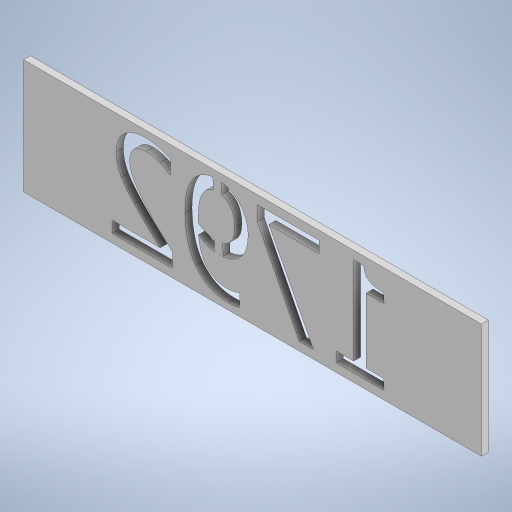
# Autodesk Inventor part: 1792 plate
Saved by Autodesk Inventor 2023.4 (Build 274418000, 418)
## iProperties
Created: 2023-12-26
Part Number: 1792 plate
Material: Generic
Document SubType Name: Sheet Metal
Designer: amrom
Density: 1 g/cm^3
Sheet Metal Rule: Default
Appearance: Default
Author: amrom
Autodesk Inventor part; units mm, degrees
ref_plane "YZ Plane" through (0, 0, 0) normal (1, 0, 0) x (0, 1, 0)
ref_plane "XZ Plane" through (0, 0, 0) normal (0, 1, 0) x (-1, 0, 0)
ref_plane "XY Plane" through (0, 0, 0) normal (0, 0, 1) x (1, 0, 0)
sketch "Sketch1" plane through (0, 0, 0) normal (0, 0, 1) x (1, 0, 0)
  line L0 (0, 0) -> (203.2, 0)
  line L1 (203.2, 0) -> (203.2, 50.8)
  line L2 (203.2, 50.8) -> (0, 50.8)
  line L3 (0, 50.8) -> (0, 0)
  dimension "d0" = 203.2
  dimension "d1" = 50.8
  measures "d0" distance of L2.end L1.end
  measures "d1" distance of L0.end L1.end
extrude "Plate1" add sketch "Sketch1" along normal blind 3.048
sketch "Sketch2" plane through (0, 0, 0) normal (0, 0, -1) x (-1, 0, 0)
  line L0 (-203.2, 0) -> (-203.2, 50.8) projected
  line L1 (-203.2, 50.8) -> (0, 50.8) projected
  line L2 (0, 0) -> (-203.2, 0) projected
  line L3 (0, 50.8) -> (0, 0) projected
  line L4 (-203.2, 50.8) -> (0, 50.8) projected
  line L5 (-203.2, 0) -> (-203.2, 50.8) projected
  line L6 (-138.7964, 3.81) -> (-159.8615, 3.81)
  line L7 (-159.8615, 3.81) -> (-159.8615, 8.219)
  line L8 (-159.8615, 8.219) -> (-152.0233, 8.219)
  line L9 (-152.0233, 8.219) -> (-152.0233, 37.1573)
  line L10 (-152.0233, 37.1573) -> (-159.8615, 37.1573)
  line L11 (-159.8615, 37.1573) -> (-159.8615, 41.1114)
  spline S0 degree 2 poles (-159.8615, 41.1114) (-155.4175, 41.1114) (-151.2185, 43.6308) (-150.9386, 47.13) knots 0 0 0 1 2 2 2
  line L12 (-150.9386, 47.13) -> (-146.4596, 47.13)
  line L13 (-146.4596, 47.13) -> (-146.4596, 8.219)
  line L14 (-146.4596, 8.219) -> (-138.7964, 8.219)
  line L15 (-138.7964, 8.219) -> (-138.7964, 3.81)
  line L16 (-103.7345, 40.5165) -> (-122.4202, 3.81)
  line L17 (-122.4202, 3.81) -> (-128.5788, 3.81)
  line L18 (-128.5788, 3.81) -> (-108.8433, 41.9162)
  line L19 (-108.8433, 41.9162) -> (-131.1332, 41.9162)
  line L20 (-131.1332, 41.9162) -> (-131.1332, 46.99)
  line L21 (-131.1332, 46.99) -> (-103.7345, 46.99)
  line L22 (-103.7345, 46.99) -> (-103.7345, 40.5165)
  spline S1 degree 2 poles (-99.6405, 32.9582) (-99.6405, 36.2825) (-97.471, 41.8112) (-95.5814, 43.8057) knots 0 0 0 1 2 2 2
  spline S2 degree 2 poles (-95.5814, 43.8057) (-93.7968, 45.7303) (-88.583, 47.8648) (-85.9236, 47.8648) knots 0 0 0 1 2 2 2
  spline S3 degree 2 poles (-85.9236, 47.8648) (-82.9493, 47.8648) (-78.1204, 45.8703) (-76.3359, 43.9807) knots 0 0 0 1 2 2 2
  spline S4 degree 2 poles (-76.3359, 43.9807) (-74.0964, 41.6012) (-71.6469, 33.903) (-71.6469, 27.9894) knots 0 0 0 1 2 2 2
  spline S5 degree 2 poles (-71.6469, 27.9894) (-71.6469, 22.6356) (-74.0614, 13.0479) (-76.4058, 9.8636) knots 0 0 0 1 2 2 2
  spline S6 degree 2 poles (-76.4058, 9.8636) (-78.8903, 6.5044) (-85.8886, 2.9702) (-90.9975, 2.9702) knots 0 0 0 1 2 2 2
  spline S7 degree 2 poles (-90.9975, 2.9702) (-92.1522, 2.9702) (-94.7766, 3.2151) (-95.8963, 3.5651) knots 0 0 0 1 2 2 2
  line L23 (-95.8963, 3.5651) -> (-95.8963, 9.1288)
  line L24 (-95.8963, 9.1288) -> (-95.6164, 9.1288)
  spline S8 degree 2 poles (-95.6164, 9.1288) (-94.8816, 8.7089) (-91.8023, 7.974) (-90.2276, 7.974) knots 0 0 0 1 2 2 2
  spline S9 degree 2 poles (-90.2276, 7.974) (-84.5589, 7.974) (-78.0854, 15.4623) (-77.6306, 22.3907) knots 0 0 0 1 2 2 2
  spline S10 degree 2 poles (-77.6306, 22.3907) (-79.94, 20.8161) (-84.139, 19.3814) (-86.6235, 19.3814) knots 0 0 0 1 2 2 2
  spline S11 degree 2 poles (-86.6235, 19.3814) (-89.0029, 19.3814) (-92.957, 20.4312) (-94.9515, 21.9358) knots 0 0 0 1 2 2 2
  spline S12 degree 2 poles (-94.9515, 21.9358) (-97.261, 23.7204) (-99.6405, 29.1441) (-99.6405, 32.9582) knots 0 0 0 1 2 2 2
  spline S13 degree 2 poles (-77.4906, 29.2841) (-77.4906, 33.6581) (-79.1002, 39.1868) (-80.5349, 40.6915) knots 0 0 0 1 2 2 2
  spline S14 degree 2 poles (-80.5349, 40.6915) (-81.7946, 42.0911) (-84.419, 43.1409) (-85.9586, 43.1409) knots 0 0 0 1 2 2 2
  spline S15 degree 2 poles (-85.9586, 43.1409) (-89.5278, 43.1409) (-93.7618, 38.0321) (-93.7618, 33.2032) knots 0 0 0 1 2 2 2
  spline S16 degree 2 poles (-93.7618, 33.2032) (-93.7618, 30.4738) (-92.3621, 26.9396) (-90.8225, 25.6799) knots 0 0 0 1 2 2 2
  spline S17 degree 2 poles (-90.8225, 25.6799) (-89.7028, 24.7701) (-86.9384, 24.1753) (-85.3288, 24.1753) knots 0 0 0 1 2 2 2
  spline S18 degree 2 poles (-85.3288, 24.1753) (-83.4742, 24.1753) (-79.2052, 25.47) (-77.5956, 26.5547) knots 0 0 0 1 2 2 2
  spline S19 degree 2 poles (-77.5956, 26.5547) (-77.5606, 26.9746) (-77.4906, 28.4093) (-77.4906, 29.2841) knots 0 0 0 1 2 2 2
  line L25 (-39.4194, 3.81) -> (-66.0482, 3.81)
  line L26 (-66.0482, 3.81) -> (-66.0482, 9.9336)
  spline S20 degree 2 poles (-66.0482, 9.9336) (-63.1789, 12.628) (-58.0701, 17.6318) (-55.6207, 20.3262) knots 0 0 0 1 2 2 2
  spline S21 degree 2 poles (-55.6207, 20.3262) (-50.6868, 25.7499) (-47.0826, 32.2584) (-47.0826, 35.7226) knots 0 0 0 1 2 2 2
  spline S22 degree 2 poles (-47.0826, 35.7226) (-47.0826, 37.5422) (-48.2024, 40.2716) (-49.2171, 41.1464) knots 0 0 0 1 2 2 2
  spline S23 degree 2 poles (-49.2171, 41.1464) (-50.2319, 42.0211) (-52.8913, 42.8959) (-54.5009, 42.8959) knots 0 0 0 1 2 2 2
  spline S24 degree 2 poles (-54.5009, 42.8959) (-56.0406, 42.8959) (-59.1898, 42.1261) (-60.6245, 41.5313) knots 0 0 0 1 2 2 2
  spline S25 degree 2 poles (-60.6245, 41.5313) (-61.8492, 41.0414) (-64.1237, 39.6417) (-64.8235, 39.1518) knots 0 0 0 1 2 2 2
  line L27 (-64.8235, 39.1518) -> (-65.1384, 39.1518)
  line L28 (-65.1384, 39.1518) -> (-65.1384, 45.3104)
  spline S26 degree 2 poles (-65.1384, 45.3104) (-63.3539, 46.1852) (-56.9503, 47.8998) (-54.081, 47.8998) knots 0 0 0 1 2 2 2
  spline S27 degree 2 poles (-54.081, 47.8998) (-48.0274, 47.8998) (-41.204, 41.4963) (-41.204, 36.0375) knots 0 0 0 1 2 2 2
  spline S28 degree 2 poles (-41.204, 36.0375) (-41.204, 33.4831) (-42.3937, 29.2141) (-43.4435, 27.3945) knots 0 0 0 1 2 2 2
  spline S29 degree 2 poles (-43.4435, 27.3945) (-44.4932, 25.505) (-47.5375, 21.7958) (-49.2171, 20.0112) knots 0 0 0 1 2 2 2
  spline S30 degree 2 poles (-49.2171, 20.0112) (-51.9465, 17.0369) (-58.63, 10.6684) (-60.6245, 8.8138) knots 0 0 0 1 2 2 2
  line L29 (-60.6245, 8.8138) -> (-39.4194, 8.8138)
  line L30 (-39.4194, 8.8138) -> (-39.4194, 3.81)
  constraints: 1 horizontal
extrude "Extrusion1" cut sketch "Sketch2" against normal blind 25.4 contours L6 L7 L8 L9 L10 L11 S0 L12 L13 L14 L15 | L16 L17 L18 L19 L20 L21 L22 | S1 S2 S3 S4 S5 S6 S7 L23 L24 S8 S9 S10 S11 S12 | L25 L26 S20 S21 S22 S23 S24 S25 L27 L28 S26 S27 S28 S29 S30 L29 L30
sketch "Sketch3" plane through (0, 0, 0) normal (0, 0, -1) x (-1, 0, 0)
  spline S0 degree 2 poles (-80.5349, 40.6915) (-81.7946, 42.0911) (-84.419, 43.1409) (-85.9586, 43.1409) knots 0 0 0 0.5 1 1 1 projected
  spline S1 degree 2 poles (-85.9586, 43.1409) (-89.5278, 43.1409) (-93.7618, 38.0321) (-93.7618, 33.2032) knots 0 0 0 0.5 1 1 1 projected
  spline S2 degree 2 poles (-90.8225, 25.6799) (-89.7028, 24.7701) (-86.9384, 24.1753) (-85.3288, 24.1753) knots 0 0 0 0.5 1 1 1 projected
  spline S3 degree 2 poles (-85.3288, 24.1753) (-83.4742, 24.1753) (-79.2052, 25.47) (-77.5956, 26.5547) knots 0 0 0 0.5 1 1 1 projected
  line L0 (0, 0) -> (-203.2, 0) projected
  line L1 (0, 50.8) -> (0, 0) projected
  line L2 (-203.2, 50.8) -> (0, 50.8) projected
  line L3 (-203.2, 0) -> (-203.2, 50.8) projected
  line L4 (-39.4194, 8.8138) -> (-39.4194, 3.81) projected
  line L5 (-39.4194, 3.81) -> (-66.0482, 3.81) projected
  line L6 (-66.0482, 3.81) -> (-66.0482, 9.9336) projected
  line L7 (-64.8235, 39.1518) -> (-65.1384, 39.1518) projected
  line L8 (-65.1384, 39.1518) -> (-65.1384, 45.3104) projected
  line L9 (-60.6245, 8.8138) -> (-39.4194, 8.8138) projected
  spline S4 degree 2 poles (-95.5814, 43.8057) (-93.7968, 45.7303) (-88.583, 47.8648) (-85.9236, 47.8648) knots 0 0 0 0.5 1 1 1 projected
  spline S5 degree 2 poles (-85.9236, 47.8648) (-82.9493, 47.8648) (-78.1204, 45.8703) (-76.3377, 43.979) knots 0 0 0 0.5 1 1 1 projected
  line L10 (-95.8963, 3.5651) -> (-95.8963, 9.1288) projected
  line L11 (-95.8963, 9.1288) -> (-95.6164, 9.1288) projected
  spline S6 degree 2 poles (-77.6306, 22.3907) (-79.94, 20.8161) (-84.139, 19.3814) (-86.6235, 19.3814) knots 0 0 0 0.5 1 1 1 projected
  spline S7 degree 2 poles (-86.6235, 19.3814) (-89.0029, 19.3814) (-92.957, 20.4312) (-94.9515, 21.9358) knots 0 0 0 0.5 1 1 1 projected
  line L12 (-138.7964, 8.219) -> (-138.7964, 3.81) projected
  line L13 (-138.7964, 3.81) -> (-159.8615, 3.81) projected
  line L14 (-159.8615, 3.81) -> (-159.8615, 8.219) projected
  line L15 (-159.8615, 8.219) -> (-152.0233, 8.219) projected
  line L16 (-152.0233, 8.219) -> (-152.0233, 37.1573) projected
  line L17 (-152.0233, 37.1573) -> (-159.8615, 37.1573) projected
  line L18 (-159.8615, 37.1573) -> (-159.8615, 41.1114) projected
  line L19 (-150.9386, 47.13) -> (-146.4596, 47.13) projected
  line L20 (-146.4596, 47.13) -> (-146.4596, 8.219) projected
  line L21 (-146.4596, 8.219) -> (-138.7964, 8.219) projected
  line L22 (-103.7345, 46.99) -> (-103.7345, 40.5165) projected
  line L23 (-103.7345, 40.5165) -> (-122.4202, 3.81) projected
  line L24 (-122.4202, 3.81) -> (-128.5788, 3.81) projected
  line L25 (-128.5788, 3.81) -> (-108.8433, 41.9162) projected
  line L26 (-108.8433, 41.9162) -> (-131.1332, 41.9162) projected
  line L27 (-131.1332, 41.9162) -> (-131.1332, 46.99) projected
  line L28 (-131.1332, 46.99) -> (-103.7345, 46.99) projected
  line L29 (-87.1345, 76.3951) -> (-88.5342, 19.4283)
  line L30 (-88.5342, 19.4283) -> (-84.7128, 19.3344)
  line L31 (-84.7128, 19.3344) -> (-83.3131, 76.3013)
  line L32 (-83.3131, 76.3013) -> (-87.1345, 76.3951)
  line L33 (-87.1345, 76.3951) -> (-84.7128, 19.3344) construction
  line L34 (-88.5342, 19.4283) -> (-83.3131, 76.3013) construction
  point P0 (-84.7088, 19.4948)
  point P1 (-84.5932, 24.2)
  point P2 (-88.4097, 24.4926)
  point P3 (-88.5331, 19.4722)
  point P4 (-87.6448, 19.4065)
  point P5 (-86.6235, 19.3814)
  point P6 (-84.1328, 42.9382)
  point P7 (-84.0145, 47.7554)
  point P8 (-87.8389, 47.7254)
  point P9 (-87.9571, 42.914)
  dimension "d5" = 3.8225
  dimension "d6" = 6.9756
  dimension "d7" = 10.1241
  constraints: 12 end point, 2 midpoint, 2 parallel, 1 perpendicular, 31 other
  measures "d5" distance between parallel lines of L31 L29
  measures "d6" distance from line of point (-77.491, 29.284) L31
  measures "d7" distance from line of point (-77.491, 29.284) L30
extrude "Extrusion2" add sketch "Sketch3" against normal up to surface (3.048 mm away) contours S0 S1 L29 S4 S5 L31 | L31 S6 L30 S7 L29 S2 S3
equation "\"d2\" = Thickness"
equation "\"BendRadius\" = Thickness"
equation "\"BendReliefWidth\" = Thickness"
equation "\"BendReliefDepth\" = 0.5 * Thickness"
equation "\"CornerReliefSize\" = 4 * Thickness"
equation "\"MinimumRemnant\" = 2 * Thickness"
equation "\"TransitionRadius\" = BendRadius"
equation "\"JacobiRadiusSize\" = BendRadius"
equation "\"GapSize\" = Thickness"
equation "\"Thickness\" = 3.048"
body "Solid1"
